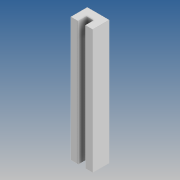
# Autodesk Inventor part: 2208_Back Plate Groove_V1
Saved by Autodesk Inventor 2020 (Build 240168000, 168)
## iProperties
Created: 2020-01-15
Part Number: 2208_Back Plate Groove_V1
Material: Generic
Document SubType Name: Modeling
Designer: RFLab
Density: 1 g/cm^3
Appearance: Default
Author: RFLab
Autodesk Inventor part; units mm, degrees
ref_plane "YZ Plane" through (0, 0, 0) normal (1, 0, 0) x (0, 1, 0)
ref_plane "XZ Plane" through (0, 0, 0) normal (0, 1, 0) x (-1, 0, 0)
ref_plane "XY Plane" through (0, 0, 0) normal (0, 0, 1) x (1, 0, 0)
sketch "Sketch1" plane through (0, 0, 0) normal (0, 0, 1) x (1, 0, 0)
  line L0 (-10, 56.825) -> (10, 56.825)
  line L1 (10, 56.825) -> (10, -56.825)
  line L2 (10, -56.825) -> (-10, -56.825)
  line L3 (-10, -56.825) -> (-10, 56.825)
  point P0 (0, 0)
  dimension "d0" = 113.65
  dimension "d1" = 56.825
  dimension "d2" = 20
  dimension "d3" = 10
  constraints: 8 end point, 2 parallel, 1 horizontal, 1 perpendicular
  measures "d0" distance of L0.end L1.end
  measures "d1" distance from line of L0 point (0, 0)
  measures "d2" distance of L0.start L0.end
  measures "d3" distance from line of L1 point (0, 0)
extrude "Extrusion1" add sketch "Sketch1" along normal blind 15
sketch "Sketch2" plane through (0, 0, 15) normal (0, 0, 1) x (1, 0, 0)
  line L0 (-10, -56.825) -> (10, -56.825) projected
  line L1 (-3.25, 56.825) -> (3.25, 56.825)
  line L2 (3.25, 56.825) -> (3.25, -56.825)
  line L3 (3.25, -56.825) -> (-3.25, -56.825)
  line L4 (-3.25, -56.825) -> (-3.25, 56.825)
  line L5 (-10, 56.825) -> (-10, -56.825) projected
  line L6 (10, -56.825) -> (10, 56.825) projected
  point P0 (0, 0)
  dimension "d6" = 6.75
  dimension "d7" = 6.5
  dimension "d8" = 20
  constraints: 8 end point, 2 parallel, 1 horizontal, 1 perpendicular, 1 point on line
  measures "d6" distance between parallel lines of L5 L4
  measures "d7" distance between parallel lines of L2 L4
  measures "d8" distance between parallel lines of L6 L5
extrude "Extrusion2" cut sketch "Sketch2" against normal blind 7.5
equation "\"d1\" = 0.5 * d0"
equation "\"d3\" = 0.5 * d2"
equation "\"d6\" = -0.5 * d7 + 0.5 * d8"
body "Solid1"
